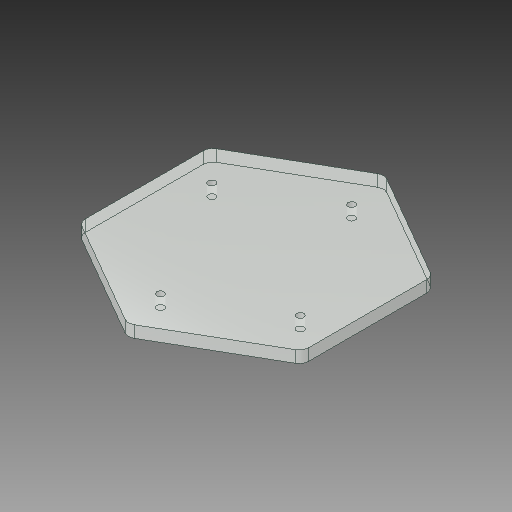
# Autodesk Inventor part: tapa
Saved by Autodesk Inventor 2018 (Build 220112000, 112)
## iProperties
Created: 2017-06-21
Part Number: tapa
Material: Generic
Document SubType Name: Modeling
Designer: Vidal Villegas
Density: 1 g/cm^3
Appearance: Clear
Mass: 38.841 g
Surface Area: 173.624 cm^2
Volume: 38.841 cm^3
Author: Vidal Villegas
Autodesk Inventor part; units mm, degrees
ref_plane "YZ Plane" through (0, 0, 0) normal (1, 0, 0) x (0, 1, 0)
ref_plane "XZ Plane" through (0, 0, 0) normal (0, 1, 0) x (-1, 0, 0)
ref_plane "XY Plane" through (0, 0, 0) normal (0, 0, 1) x (1, 0, 0)
sketch "Sketch1" plane through (0, 0, 0) normal (0, 1, 0) x (-1, 0, 0)
  line L0 (-47.5136, -27.432) -> (-47.5136, 27.432)
  line L1 (-47.5136, 27.432) -> (0, 54.864)
  line L2 (0, 54.864) -> (47.5136, 27.432)
  line L3 (47.5136, 27.432) -> (47.5136, -27.432)
  line L4 (47.5136, -27.432) -> (0, -54.864)
  line L5 (0, -54.864) -> (-47.5136, -27.432)
  line L6 (0, 54.864) -> (47.5136, 27.432)
  line L7 (47.5136, 27.432) -> (47.5136, -27.432)
  line L8 (47.5136, -27.432) -> (0, -54.864)
  line L9 (0, -54.864) -> (-47.5136, -27.432)
  line L10 (-47.5136, -27.432) -> (-47.5136, 27.432)
  line L11 (-47.5136, 27.432) -> (0, 54.864)
  line L12 (0, 54.805) -> (-47.4625, 27.4025)
  line L13 (-47.4625, 27.4025) -> (-47.4625, -27.4025)
  line L14 (-47.4625, -27.4025) -> (0, -54.805)
  line L15 (-47.4625, 27.4025) -> (0, 54.805)
  line L16 (0, 54.805) -> (47.4625, 27.4025)
  line L17 (47.4625, 27.4025) -> (47.4625, -27.4025)
  line L18 (47.4625, -27.4025) -> (0, -54.805)
  line L19 (0, -54.805) -> (-47.4625, -27.4025)
  line L20 (-47.4625, -27.4025) -> (-47.4625, 27.4025)
  circle A0 centre (-33.775, 15) radius 1.55
  circle A1 centre (-3.8971, -36.75) radius 1.55
  circle A2 centre (33.775, -15) radius 1.55
  circle A3 centre (3.8971, 36.75) radius 1.55
  line L21 (-33.775, 19.5) -> (0, 39) construction
  line L22 (0, 39) -> (33.775, 19.5) construction
  line L23 (33.775, 19.5) -> (33.775, -19.5) construction
  line L24 (33.775, -19.5) -> (0, -39) construction
  line L25 (0, -39) -> (-33.775, -19.5) construction
  line L26 (-33.775, -19.5) -> (-33.775, 19.5) construction
  line L27 (-44.5136, -25.6999) -> (-44.5136, 25.6999)
  line L28 (-44.5136, 25.6999) -> (0, 51.3999)
  line L29 (0, 51.3999) -> (44.5136, 25.6999)
  line L30 (44.5136, 25.6999) -> (44.5136, -25.6999)
  line L31 (0, -51.3999) -> (-44.5136, -25.6999)
  line L32 (47.5136, -27.432) -> (47.5136, 27.432)
  line L33 (47.5136, 27.432) -> (0, 54.864)
  line L34 (0, 54.864) -> (-47.5136, 27.432)
  line L35 (-47.5136, 27.432) -> (-47.5136, -27.432)
  line L36 (-47.5136, -27.432) -> (0, -54.864)
  line L37 (0, -54.864) -> (47.5136, -27.432)
  line L38 (44.5136, 25.6999) -> (44.5136, -25.6999)
  line L39 (29.2636, 11) -> (29.2636, -11)
  line L40 (44.5136, -11) -> (44.5136, 11)
  line L41 (44.5136, 0) -> (46.3422, 0) construction
  line L42 (0, -33.7907) -> (-29.2636, -16.8954) construction
  line L43 (-29.2636, -16.8954) -> (-29.2636, 16.8954) construction
  line L44 (-29.2636, 16.8954) -> (-16.4566, 24.2895) construction
  line L45 (0, 33.7907) -> (29.2636, 16.8954) construction
  line L46 (29.2636, 16.8954) -> (29.2636, -16.8954) construction
  line L47 (29.2636, -16.8954) -> (16.4566, -24.2895) construction
  line L48 (0, -51.3999) -> (-44.5136, -25.6999) construction
  line L49 (20.432, -39.6035) -> (0, -51.3999) construction
  line L50 (44.5136, -25.6999) -> (24.0816, -37.4964) construction
  line L51 (44.5136, 25.6999) -> (44.5136, -25.6999) construction
  line L52 (0, 51.3999) -> (44.5136, 25.6999) construction
  line L53 (-20.432, 39.6035) -> (0, 51.3999) construction
  line L54 (-44.5136, 25.6999) -> (-24.0816, 37.4964) construction
  line L55 (-44.5136, -25.6999) -> (-44.5136, 25.6999) construction
  line L56 (29.2636, 16.8954) -> (0, 33.7907)
  line L57 (31.7831, 33.0499) -> (12.7305, 44.0499)
  line L58 (22.2568, 38.5499) -> (22.6365, 39.2076)
  line L59 (0, 51.3999) -> (44.5136, 25.6999)
  line L60 (0, 33.7907) -> (29.2636, 16.8954)
  line L61 (0, 0) -> (0, -5.712) construction
  line L62 (0, 0) -> (4.8403, -2.7945) construction
  line L63 (29.2636, 16.8954) -> (29.2636, -16.8954) construction
  line L64 (-44.5136, -11) -> (-44.5136, 11)
  line L65 (-22.2568, -38.5499) -> (-22.6365, -39.2076)
  line L66 (-12.7305, -44.0499) -> (-31.7831, -33.0499)
  line L67 (-24.1581, -19.843) -> (-5.1055, -30.843)
  line L68 (0, -54.864) -> (47.5136, -27.432) construction
  line L69 (23.7568, -41.148) -> (25.1641, -43.5855) construction
  line L70 (29.2636, -16.8954) -> (0, -33.7907)
  line L71 (0, 0) -> (6.6102, 3.8164) construction
  line L72 (0, 51.3999) -> (-44.5136, 25.6999)
  line L73 (0, 33.7907) -> (-29.2636, 16.8954) construction
  line L74 (-24.1581, 19.843) -> (-31.7831, 33.0499)
  line L75 (-31.7831, 33.0499) -> (-12.7305, 44.0499)
  line L76 (5.1055, -30.843) -> (24.1581, -19.843)
  line L77 (0, -33.7907) -> (29.2636, -16.8954)
  line L78 (41.3094, 27.5499) -> (29.4425, 34.4013)
  line L79 (31.7831, 33.0499) -> (12.7305, 44.0499)
  line L80 (-12.7305, 44.0499) -> (-31.7831, 33.0499)
  line L81 (-31.7831, 33.0499) -> (-24.1581, 19.843)
  line L82 (-5.1055, -30.843) -> (-24.1581, -19.843)
  line L83 (0, -33.7907) -> (-29.2636, -16.8954)
  line L84 (-31.7831, -33.0499) -> (-12.7305, -44.0499)
  line L85 (12.807, -26.3966) -> (0, -33.7907)
  line L86 (-12.807, 26.3966) -> (0, 33.7907)
  point P0 (-44.5136, 0)
  point P1 (-44.5136, 0)
  dimension "d0" = 54.864
  dimension "d1" = 0
  dimension "d3" = 39
  dimension "d6" = 4.5
  dimension "d7" = 4.5
  dimension "d11" = 4.5
  dimension "d15" = 4.5
  constraints: 174 end point, 9 point on line, 9 symmetric about line, 6 coincident, 4 centre point, 4 collinear, 4 parallel, 3 perpendicular, 3 vertical, 3 vertical alignment, 1 horizontal, 1 midpoint, 52 other
  measures "d0" distance of L0.start L0.end
  measures "d1" distance between parallel lines of L1 L11
  measures "d3" distance of L26.start L21.start
  measures "d6" distance of L21.start A0.centre
  measures "d7" distance of A1.centre L24.end
  measures "d11" distance of A3.centre L21.end
  measures "d15" distance of A2.centre L23.end
extrude "Extrusion2" add sketch "Sketch1" along normal blind 5 contours L16 L17 L18 L14 L13 L12
fillet "Fillet1" radius 4 6 edges at (47.4625, 2.5, 27.4025) (0, 2.5, 54.805) (-47.4625, 2.5, 27.4025) (-47.4625, 2.5, -27.4025) (0, 2.5, -54.805) (47.4625, 2.5, -27.4025)
equation "\"d6\" = d4"
equation "\"d7\" = d5"
equation "\"d11\" = d4"
equation "\"d15\" = d9"
equation "\"d5\" = d4"
equation "\"d9\" = d4"
equation "\"d4\" = 4.5"
body "Solid2"
